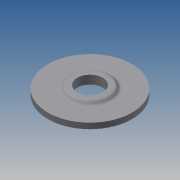
# Autodesk Inventor part: washer
Saved by Autodesk Inventor 2014 (Build 180170000, 170)
## iProperties
Created: 2014-01-25
Part Number: washer
Material: Generic
Document SubType Name: Modeling
Designer: Peele
Density: 1 g/cm^3
Appearance: Default
Author: Peele
Autodesk Inventor part; units mm, degrees
ref_plane "YZ Plane" through (0, 0, 0) normal (1, 0, 0) x (0, 1, 0)
ref_plane "XZ Plane" through (0, 0, 0) normal (0, 1, 0) x (-1, 0, 0)
ref_plane "XY Plane" through (0, 0, 0) normal (0, 0, 1) x (1, 0, 0)
sketch "Sketch1" plane through (0, 0, 0) normal (0, 1, 0) x (-1, 0, 0)
  line L0 (4.5, 0) -> (4.5, 3)
  line L1 (4.5, 3) -> (6.5, 3)
  line L2 (6.5, 3) -> (7.5, 2)
  line L3 (7.5, 2) -> (14.875, 2)
  line L4 (14.875, 2) -> (14.875, 0)
  line L5 (14.875, 0) -> (4.5, 0)
  line L6 (0, 0) -> (0, 4.9053) construction
  dimension "d0" = 14.875
  dimension "d1" = 4.5
  dimension "d2" = 6.5
  dimension "d3" = 2
  dimension "d4" = 3
  dimension "d5" = 1
  constraints: 14 end point, 3 parallel, 2 perpendicular, 1 point on line, 1 vertical
  measures "d0" distance from line of L4 L6.start
  measures "d1" distance from line of L6.start L0
  measures "d2" horizontal distance of L6.start L1.end
  measures "d3" distance of L3.end L4.end
  measures "d4" distance of L0.start L0.end
  measures "d5" horizontal distance of L1.end L2.end
revolve "Revolution1" add sketch "Sketch1" angle 360 about axis through (0, 0, 0) along (0, 0, 1)
fillet "Fillet1" radius 1 2 edges at (7.5, 0, 2) (6.5, 0, 3)
body "Solid1"
